Autodesk Fusion 360 part; units mm, degrees
note: some values were not read from the file. Chosen so that the rebuilt part matches the saved one: which bodies a step acts on; a direction; that a step has no effect; which face or edge a step refers to; which pieces of a blend or face edit are solid. Set by a fixed rule: which sketch regions a step uses.
(part 3 of 3)
chamfer "Fase5" distance 4 distance2 4.7 5 edges at (117, 33.2, 162.2) (55.5, 33.2, 162.2) (-2, 33.2, 162.2) (122, 87.4, 162.2) (-7, 87.4, 162.2) measured on face at (116.9689, 33.2, 167.6178) measured on face at (55.5311, 33.2, 167.6512) measured on face at (-1.9689, 33.2, 167.6178) measured on face at (122, 89.0667, 124.4667) measured on face at (-7, 85.7333, 101.1333) on bodies 16
chamfer "Fase6" distance 3 distance2 2.4 5 edges at (-2, 30.8, 202.2) (55.5, 30.8, 202.2) (117, 30.8, 202.2) (122, 87.4, 202.2) (-7, 87.4, 202.2) measured on face at (-3.6667, 30.8, 197.2) measured on face at (55.5311, 30.8, 195.1488) measured on face at (118.6667, 30.8, 197.2) measured on face at (122, 85.7333, 250.1333) measured on face at (-7, 85.7333, 284.4) on bodies 12
sketch "Skizze25" plane through (0, 0, -160.2) normal (0, 0, -1) x (-1, 0, 0)
  line L0 (9.4, 0) -> (9.4, 90)
  line L1 (-97.8, 90) -> (-185, 90)
  line L2 (-185, 90) -> (-185, 0)
  line L3 (-175, 47) -> (-1.2, 47)
  line L4 (-1.2, 47) -> (-1.2, 40)
  line L5 (-1.2, 40) -> (-175, 40)
  line L6 (-175, 40) -> (-175, 47)
  line L7 (-175, 50) -> (-1.2, 50)
  line L8 (-1.2, 50) -> (-1.2, 57)
  line L9 (-1.2, 57) -> (-175, 57)
  line L10 (-175, 57) -> (-175, 50)
  line L11 (-175, 60) -> (-1.2, 60)
  line L12 (-1.2, 60) -> (-1.2, 67)
  line L13 (-1.2, 67) -> (-175, 67)
  line L14 (-175, 67) -> (-175, 60)
  line L15 (-175, 70) -> (-1.2, 70)
  line L16 (-1.2, 70) -> (-1.2, 77)
  line L17 (-1.2, 77) -> (-175, 77)
  line L18 (-175, 77) -> (-175, 70)
  line L19 (-175, 80) -> (-1.2, 80)
  line L20 (-1.2, 80) -> (-1.2, 87)
  line L21 (-1.2, 87) -> (-175, 87)
  line L22 (-175, 87) -> (-175, 80)
  line L23 (-86.6, 87) -> (-89.6, 87)
  line L24 (-89.6, 87) -> (-89.6, 10)
  line L25 (-86.6, 10) -> (-86.6, 87)
  line L26 (8.8, 91.8) -> (8.8, 0)
  line L27 (-67.35, 22) -> (-50.9, 22)
  line L28 (-50.9, 22) -> (-50.9, 10)
  line L29 (-50.9, 10) -> (-67.35, 10)
  line L30 (-67.35, 10) -> (-67.35, 22)
  line L31 (-48.9, 10) -> (-48.9, 20)
  line L32 (-48.9, 20) -> (-31.68, 20)
  line L33 (-31.68, 20) -> (-31.68, 10)
  line L34 (-84.55, 10) -> (-84.55, 25)
  line L35 (-84.55, 25) -> (-69.35, 25)
  line L36 (-69.35, 25) -> (-69.35, 10)
  line L37 (-185, 0) -> (9.4, 0)
  line L38 (-175, 30) -> (-175, 37)
  line L39 (-1.2, 30) -> (-175, 30)
  line L40 (-84.55, 15) -> (-69.35, 15)
  line L41 (-175, 37) -> (-1.2, 37)
  line L42 (-1.2, 37) -> (-1.2, 30)
  line L43 (-89.6, 30) -> (-86.6, 30)
  line L44 (-175, 20) -> (-175, 27)
  line L45 (-1.2, 20) -> (-175, 20)
  line L46 (-84.55, 5) -> (-69.35, 5)
  line L47 (-175, 27) -> (-1.2, 27)
  line L48 (-1.2, 27) -> (-1.2, 20)
  line L49 (-89.6, 20) -> (-86.6, 20)
  line L50 (-175, 10) -> (-175, 17)
  line L51 (-1.2, 10) -> (-175, 10)
  line L52 (-84.55, -5) -> (-69.35, -5)
  line L53 (-175, 17) -> (-1.2, 17)
  line L54 (-1.2, 17) -> (-1.2, 10)
  line L55 (-89.6, 10) -> (-86.6, 10)
  line L56 (-56.3, 0) -> (-58.3, 0)
  line L57 (-58.3, 0) -> (-58.3, 47.5)
  line L58 (-58.3, 47.5) -> (-56.3, 47.5)
  line L59 (-56.3, 47.5) -> (-56.3, 0)
  line L60 (-58.3, 0) -> (-61.3, 0)
  line L61 (-61.3, 0) -> (-61.3, 47.5)
  line L62 (-61.3, 47.5) -> (-58.3, 47.5)
  line L63 (-58.3, 47.5) -> (-58.3, 0)
  line L64 (-56.3, 0) -> (-53.3, 0)
  line L65 (-53.3, 0) -> (-53.3, 49.9654)
  line L66 (-53.3, 49.9654) -> (-56.3, 49.9654)
  line L67 (-56.3, 49.9654) -> (-56.3, 0)
  line L68 (8.8, 0) -> (-122.3, 0)
  line L69 (-42.3, 57) -> (-42.3, 40)
  line L70 (-77.8, 90) -> (-77.8, 99)
  line L71 (-77.8, 99) -> (-84.8, 105)
  line L72 (-84.8, 105) -> (-90.8, 105)
  line L73 (-90.8, 105) -> (-97.8, 99)
  line L74 (-97.8, 99) -> (-97.8, 90)
  line L75 (9.4, 90) -> (-10.6, 90)
  line L76 (-10.6, 90) -> (-10.6, 99)
  line L77 (-10.6, 99) -> (-17.6, 105)
  line L78 (-17.6, 105) -> (-23.6, 105)
  line L79 (-23.6, 105) -> (-30.6, 99)
  line L80 (-30.6, 99) -> (-30.6, 90)
  line L81 (-30.6, 90) -> (-77.8, 90)
  line L82 (-31.68, 10) -> (-48.9, 10)
  line L83 (-69.35, 10) -> (-84.55, 10)
  circle A0 centre (-87.8, 99) radius 2.05
  circle A1 centre (-20.6, 99) radius 2.05
  point P0 (-57.3, 47.5)
  dimension "d531" = 7
  dimension "d533" = 7
  dimension "d534" = 7
  dimension "d535" = 7
  dimension "d536" = 3
  dimension "d537" = 3
  dimension "d538" = 3
  dimension "d539" = 7
  dimension "d540" = 3
  dimension "d541" = 10
  dimension "d561" = 3
  dimension "d719" = 10
  dimension "d720" = 7
  dimension "d721" = 7
  dimension "d722" = 7
  dimension "d723" = 3
  dimension "d724" = 3
  dimension "d725" = 3
  dimension "d726" = 2
  dimension "d727" = 3
  dimension "d728" = 3
  dimension "d753" = 15
  constraint horizontal L3
  constraint vertical L4
  constraint horizontal L5
  constraint vertical L6
  constraint horizontal L7
  constraint vertical L8
  constraint horizontal L9
  constraint vertical L10
  constraint horizontal L11
  constraint vertical L12
  constraint horizontal L13
  constraint vertical L14
  constraint horizontal L15
  constraint vertical L16
  constraint horizontal L17
  constraint vertical L18
  constraint horizontal L19
  constraint vertical L20
  constraint horizontal L21
  constraint vertical L22
  constraint vertical L3.start L7.start
  constraint vertical L9.end L11.start
  constraint vertical L13.end L15.start
  constraint vertical L3.end L7.end
  constraint vertical L8.end L11.end
  constraint vertical L12.end L15.end
  constraint vertical L16.end L19.end
  constraint horizontal L23
  constraint vertical L24
  constraint vertical L25
  constraint coincident L21 L23.end
  constraint vertical L17.end L19.start
  constraint horizontal L41
  constraint vertical L42
  constraint horizontal L39
  constraint vertical L38
  constraint horizontal L43
  constraint midpoint L39 L43
  constraint horizontal L47
  constraint vertical L48
  constraint horizontal L45
  constraint vertical L44
  constraint horizontal L49
  constraint midpoint L45 L49
  constraint horizontal L53
  constraint vertical L54
  constraint horizontal L51
  constraint vertical L50
  constraint horizontal L55
  constraint midpoint L51 L55
  constraint horizontal L56
  constraint vertical L57
  constraint horizontal L58
  constraint vertical L59
  constraint coincident L37 L56.start
  constraint midpoint L58 P0
  constraint horizontal L60
  constraint vertical L61
  constraint horizontal L62
  constraint vertical L63
  constraint horizontal L64
  constraint vertical L65
  constraint horizontal L66
  constraint vertical L67
  constraint vertical L5.end L38.end
  constraint vertical L38.start L44.end
  constraint vertical L44.start L50.end
  constraint coincident L34.start L51
  constraint coincident L9 L69.start
  constraint coincident L5 L69.end
  constraint perpendicular L5 L69
  measures "d531" distance of L3 L5
  measures "d533" distance of L7.start L9.end
  measures "d534" distance of L11.start L13.end
  measures "d535" distance of L15.start L17.end
  measures "d536" distance of L3 L7
  measures "d537" distance of L9 L11
  measures "d538" distance of L13 L15
  measures "d539" distance of L19.start L21.end
  measures "d540" distance of L17 L19
  measures "d541" distance of L2 L22
  measures "d561" distance of L24 L25
  measures "d719" distance of L20 L26
  measures "d720" distance of L39 L41
  measures "d721" distance of L45 L47
  measures "d722" distance of L51 L53
  measures "d723" distance of L5 L41
  measures "d724" distance of L39 L47
  measures "d725" distance of L45 L53
  measures "d726" distance of L57 L59
  measures "d727" distance of L56.end L60.end
  measures "d728" distance of L56.start L64.end
  measures "d753" distance of P0 L69
sketch "Skizze26" plane through (-9.4, 0, 0) normal (-1, 0, 0) x (0, 0, 1)
  line L0 (-69.4, 90) -> (-120.2, 90)
  line L1 (-120.2, 90) -> (-120.2, 98)
  line L2 (-126.2, 105) -> (-134.2, 105)
  line L3 (-150.2, 47) -> (-39.4, 47)
  line L4 (-39.4, 47) -> (-39.4, 40)
  line L5 (-39.4, 40) -> (-150.2, 40)
  line L6 (-150.2, 40) -> (-150.2, 47)
  line L7 (-150.2, 50) -> (-39.4, 50)
  line L8 (-39.4, 50) -> (-39.4, 57)
  line L9 (-39.4, 57) -> (-150.2, 57)
  line L10 (-150.2, 57) -> (-150.2, 50)
  line L11 (-150.2, 60) -> (-39.4, 60)
  line L12 (-39.4, 60) -> (-39.4, 67)
  line L13 (-39.4, 67) -> (-150.2, 67)
  line L14 (-150.2, 67) -> (-150.2, 60)
  line L15 (-150.2, 70) -> (-39.4, 70)
  line L16 (-39.4, 70) -> (-39.4, 77)
  line L17 (-39.4, 77) -> (-150.2, 77)
  line L18 (-150.2, 77) -> (-150.2, 70)
  line L19 (-150.2, 87) -> (-39.4, 87)
  line L20 (-39.4, 87) -> (-39.4, 80)
  line L21 (-39.4, 80) -> (-150.2, 80)
  line L22 (-150.2, 80) -> (-150.2, 87)
  line L23 (-150.2, 37) -> (-39.4, 37)
  line L24 (-39.4, 37) -> (-39.4, 30)
  line L25 (-39.4, 30) -> (-150.2, 30)
  line L26 (-150.2, 30) -> (-150.2, 37)
  line L27 (-150.2, 27) -> (-39.4, 27)
  line L28 (-39.4, 27) -> (-39.4, 20)
  line L29 (-39.4, 20) -> (-150.2, 20)
  line L30 (-150.2, 20) -> (-150.2, 27)
  line L31 (-96.3, 87) -> (-93.3, 87)
  line L32 (-93.3, 87) -> (-93.3, 10)
  line L33 (-93.3, 10) -> (-96.3, 10)
  line L34 (-96.3, 10) -> (-96.3, 87)
  line L35 (-29.4, 185.4469) -> (-29.4, 23.7878)
  line L36 (-150.2, 17) -> (-39.4, 17)
  line L37 (-39.4, 10) -> (-150.2, 10)
  line L38 (-39.4, 17) -> (-39.4, 10)
  line L39 (-150.2, 10) -> (-150.2, 17)
  line L40 (-131.2, 38.5) -> (-129.2, 38.5)
  line L41 (-129.2, 38.5) -> (-129.2, 0)
  line L42 (-129.2, 0) -> (-131.2, 0)
  line L43 (-131.2, 0) -> (-131.2, 38.5)
  line L44 (-60.4, 0) -> (-58.4, 0)
  line L45 (-58.4, 0) -> (-58.4, 38.5)
  line L46 (-58.4, 38.5) -> (-60.4, 38.5)
  line L47 (-60.4, 38.5) -> (-60.4, 0)
  line L48 (-60.4, 38.5) -> (-63.4, 38.5)
  line L49 (-63.4, 38.5) -> (-63.4, 10)
  line L50 (-63.4, 10) -> (-60.4, 10)
  line L51 (-60.4, 10) -> (-60.4, 38.5)
  line L52 (-58.4, 38.5) -> (-55.4, 38.5)
  line L53 (-55.4, 38.5) -> (-55.4, 10)
  line L54 (-58.4, 0) -> (-58.4, 38.5)
  line L55 (-160.2, 0) -> (-160.2, 90)
  line L56 (-29.4, 0) -> (-160.2, 0)
  line L57 (-129.2, 38.5) -> (-126.2, 38.5)
  line L58 (-126.2, 38.5) -> (-126.2, 10)
  line L59 (-126.2, 10) -> (-129.2, 10)
  line L60 (-129.2, 10) -> (-129.2, 38.5)
  line L61 (-131.2, 38.5) -> (-134.2, 38.5)
  line L62 (-134.2, 38.5) -> (-134.2, 10)
  line L63 (-134.2, 10) -> (-131.2, 10)
  line L64 (-131.2, 10) -> (-131.2, 38.5)
  line L65 (-74.4, 47) -> (-113.2155, 47)
  line L66 (-113.2155, 47) -> (-113.2155, 30)
  line L67 (-113.2155, 30) -> (-74.4, 30)
  line L68 (-74.4, 30) -> (-74.4, 47)
  circle A0 centre (-59.4, 38.5) radius 10
  line L69 (-134.2, 105) -> (-140.2, 98)
  line L70 (-49.4, 98) -> (-55.4, 105)
  line L71 (-63.4, 105) -> (-69.4, 98)
  line L72 (-120.2, 98) -> (-126.2, 105)
  line L73 (-29.4, 90) -> (-49.4, 90)
  line L74 (-29.4, 0) -> (-29.4, 90)
  line L75 (-69.4, 98) -> (-69.4, 90)
  circle A1 centre (-130.2, 99) radius 2.05
  point P0 (-130.2, 38.5)
  point P1 (-59.4, 38.5)
  dimension "d542" = 7
  dimension "d545" = 7
  dimension "d546" = 7
  dimension "d547" = 7
  dimension "d548" = 3
  dimension "d549" = 3
  dimension "d550" = 3
  dimension "d551" = 7
  dimension "d552" = 3
  dimension "d553" = 7
  dimension "d556" = 3
  dimension "d557" = 3
  dimension "d559" = 7
  dimension "d560" = 3
  dimension "d730" = 10
  dimension "d731" = 7
  dimension "d732" = 3
  dimension "d738" = 2
  dimension "d739" = 2
  dimension "d741" = 3
  dimension "d743" = 3
  dimension "d744" = 10
  dimension "d745" = 10
  dimension "d749" = 3
  dimension "d750" = 3
  dimension "d751" = 15
  dimension "d752" = 16.9845
  constraint horizontal L3
  constraint vertical L4
  constraint horizontal L5
  constraint vertical L6
  constraint horizontal L7
  constraint vertical L8
  constraint horizontal L9
  constraint vertical L10
  constraint horizontal L11
  constraint vertical L12
  constraint horizontal L13
  constraint vertical L14
  constraint horizontal L15
  constraint vertical L16
  constraint horizontal L17
  constraint vertical L18
  constraint horizontal L19
  constraint vertical L20
  constraint horizontal L21
  constraint vertical L22
  constraint vertical L3.start L7.start
  constraint vertical L9.end L11.start
  constraint vertical L13.end L15.start
  constraint vertical L17.end L21.end
  constraint vertical L3.end L7.end
  constraint vertical L8.end L11.end
  constraint vertical L12.end L15.end
  constraint vertical L16.end L20.end
  constraint horizontal L23
  constraint vertical L24
  constraint horizontal L25
  constraint vertical L26
  constraint horizontal L27
  constraint vertical L28
  constraint horizontal L29
  constraint vertical L30
  constraint vertical L5.end L23.start
  constraint vertical L25.end L27.start
  constraint vertical L24.end L27.end
  constraint vertical L4.end L23.end
  constraint horizontal L31
  constraint vertical L32
  constraint horizontal L33
  constraint vertical L34
  constraint coincident L19 L31.start
  constraint midpoint L19 L31
  constraint horizontal L36
  constraint vertical L38
  constraint horizontal L37
  constraint vertical L39
  constraint coincident L32.end L37
  constraint vertical L29.end L36.start
  constraint vertical L28.end L36.end
  constraint horizontal L40
  constraint vertical L41
  constraint horizontal L42
  constraint vertical L43
  constraint midpoint L40 P0
  constraint horizontal L44
  constraint vertical L45
  constraint horizontal L46
  constraint vertical L47
  constraint midpoint L46 P1
  constraint horizontal L48
  constraint vertical L49
  constraint horizontal L50
  constraint vertical L51
  constraint horizontal L52
  constraint vertical L53
  constraint vertical L54
  constraint coincident L37 L53.end
  constraint coincident L37 L49.end
  constraint horizontal L57
  constraint vertical L58
  constraint horizontal L59
  constraint vertical L60
  constraint horizontal L61
  constraint vertical L62
  constraint horizontal L63
  constraint vertical L64
  constraint coincident L37 L62.end
  constraint coincident L37 L58.end
  constraint horizontal L65
  constraint vertical L66
  constraint horizontal L67
  constraint vertical L68
  constraint coincident L25 L66.end
  constraint coincident L3 L65.start
  constraint coincident L44.end L56
  constraint coincident L44.start L56
  constraint coincident L41.end L56
  measures "d542" distance of L3.start L5.end
  measures "d545" distance of L7.start L9.end
  measures "d546" distance of L11.start L13.end
  measures "d547" distance of L15.start L17.end
  measures "d548" distance of L3 L7
  measures "d549" distance of L9 L11
  measures "d550" distance of L13 L15.end
  measures "d551" distance of L19.start L21.end
  measures "d552" distance of L17 L21
  measures "d553" distance of L23.start L25.end
  measures "d556" distance of L5 L23
  measures "d557" distance of L25 L27
  measures "d559" distance of L27 L29
  measures "d560" distance of L32 L34
  measures "d730" distance of L20 L35
  measures "d731" distance of L36 L37
  measures "d732" distance of L29 L36
  measures "d738" distance of L41 L43
  measures "d739" distance of L45 L47
  measures "d741" distance of L46.end L48.end
  measures "d743" distance of L45.end L52.end
  measures "d744" distance of L22 L55
  measures "d745" distance of L37 L56
  measures "d749" distance of L40.end L57.end
  measures "d750" distance of L40.start L61.end
  measures "d751" distance of L68 P1
  measures "d752" distance of P0 L66
sketch "Skizze27" plane through (0, -2.4, 0) normal (0, -1, 0) x (-1, 0, 0)
  line L0 (-29.653, 141.5068) -> (-29.653, 45.5068)
  line L1 (-29.653, 45.5068) -> (-36.653, 45.5068)
  line L2 (-36.653, 141.5068) -> (-29.653, 141.5068)
  line L3 (-66.653, 45.5068) -> (-66.653, 141.5068)
  line L4 (-59.653, 45.5068) -> (-66.653, 45.5068)
  line L5 (-69.653, 45.5068) -> (-76.653, 45.5068)
  line L6 (-39.653, 45.5068) -> (-46.653, 45.5068)
  line L7 (-49.653, 45.5068) -> (-56.653, 45.5068)
  line L8 (-39.653, 141.5068) -> (-39.653, 45.5068)
  line L9 (-59.653, 141.5068) -> (-59.653, 45.5068)
  line L10 (-46.653, 45.5068) -> (-46.653, 141.5068)
  line L11 (-56.653, 45.5068) -> (-56.653, 141.5068)
  line L12 (-69.653, 141.5068) -> (-69.653, 45.5068)
  line L13 (-49.653, 141.5068) -> (-49.653, 45.5068)
  line L14 (-76.653, 45.5068) -> (-76.653, 141.5068)
  line L15 (-46.653, 141.5068) -> (-39.653, 141.5068)
  line L16 (-66.653, 141.5068) -> (-59.653, 141.5068)
  line L17 (-76.653, 141.5068) -> (-69.653, 141.5068)
  line L18 (-56.653, 141.5068) -> (-49.653, 141.5068)
  line L19 (-106.653, 45.5068) -> (-106.653, 141.5068)
  line L20 (-99.653, 45.5068) -> (-106.653, 45.5068)
  line L21 (-109.653, 45.5068) -> (-116.653, 45.5068)
  line L22 (-79.653, 45.5068) -> (-86.653, 45.5068)
  line L23 (-89.653, 45.5068) -> (-96.653, 45.5068)
  line L24 (-79.653, 141.5068) -> (-79.653, 45.5068)
  line L25 (-99.653, 141.5068) -> (-99.653, 45.5068)
  line L26 (-86.653, 45.5068) -> (-86.653, 141.5068)
  line L27 (-96.653, 45.5068) -> (-96.653, 141.5068)
  line L28 (-109.653, 141.5068) -> (-109.653, 45.5068)
  line L29 (-89.653, 141.5068) -> (-89.653, 45.5068)
  line L30 (-116.653, 45.5068) -> (-116.653, 141.5068)
  line L31 (-86.653, 141.5068) -> (-79.653, 141.5068)
  line L32 (-106.653, 141.5068) -> (-99.653, 141.5068)
  line L33 (-116.653, 141.5068) -> (-109.653, 141.5068)
  line L34 (-96.653, 141.5068) -> (-89.653, 141.5068)
  line L35 (-146.653, 45.5068) -> (-146.653, 141.5068)
  line L36 (-139.653, 45.5068) -> (-146.653, 45.5068)
  line L37 (-161.653, 45.5068) -> (-168.653, 45.5068)
  line L38 (-119.653, 45.5068) -> (-126.653, 45.5068)
  line L39 (-129.653, 45.5068) -> (-136.653, 45.5068)
  line L40 (-119.653, 141.5068) -> (-119.653, 45.5068)
  line L41 (-139.653, 141.5068) -> (-139.653, 45.5068)
  line L42 (-126.653, 45.5068) -> (-126.653, 141.5068)
  line L43 (-136.653, 45.5068) -> (-136.653, 141.5068)
  line L44 (-161.653, 141.5068) -> (-161.653, 45.5068)
  line L45 (-129.653, 141.5068) -> (-129.653, 45.5068)
  line L46 (-168.653, 45.5068) -> (-168.653, 141.5068)
  line L47 (-126.653, 141.5068) -> (-119.653, 141.5068)
  line L48 (-146.653, 141.5068) -> (-139.653, 141.5068)
  line L49 (-168.653, 141.5068) -> (-161.653, 141.5068)
  line L50 (-136.653, 141.5068) -> (-129.653, 141.5068)
  line L51 (-36.653, 45.5068) -> (-36.653, 141.5068)
  line L52 (-178.653, 45.5068) -> (-178.653, 141.5068)
  line L53 (-171.653, 45.5068) -> (-178.653, 45.5068)
  line L54 (-171.653, 141.5068) -> (-171.653, 45.5068)
  line L55 (-178.653, 141.5068) -> (-171.653, 141.5068)
  line L56 (-29.653, 95.0068) -> (-29.653, 92.0068)
  line L57 (-29.653, 92.0068) -> (-178.653, 92.0068)
  line L58 (-178.653, 92.0068) -> (-178.653, 95.0068)
  line L59 (-178.653, 95.0068) -> (-29.653, 95.0068)
  circle A0 centre (-179.1, 154.3) radius 1.5
  circle A1 centre (3.5, 35.3) radius 1.5
  circle A2 centre (-155.5, 66.3) radius 1.5
  circle A3 centre (-17.5, 66.3) radius 1.5
  circle A4 centre (-179.1, 35.3) radius 1.5
  line L60 (2, 96.8) -> (-8, 96.8)
  line L61 (-8, 96.8) -> (-8, 116.8)
  line L62 (-8, 116.8) -> (2, 116.8)
  line L63 (2, 116.8) -> (2, 96.8)
  circle A5 centre (-17.5, 152.3) radius 1.5
  circle A6 centre (-155.5, 152.3) radius 1.5
  circle A7 centre (3.5, 154.3) radius 1.5
  line L64 (-185, 29.4) -> (9.4, 29.4)
  line L65 (9.4, 29.4) -> (9.4, 160.2)
  line L66 (9.4, 160.2) -> (-185, 160.2)
  line L67 (-185, 160.2) -> (-185, 29.4)
  line L68 (-97.8, 157.8) -> (-182.6, 157.8)
  line L69 (-30.6, 157.8) -> (-77.8, 157.8)
  line L70 (7, 157.8) -> (-10.6, 157.8)
  point P0 (-36.653, 141.5068)
  point P1 (-36.653, 45.5068)
  point P2 (-36.653, 141.5068)
  point P3 (-79.653, 143.3514)
  point P4 (-76.653, 45.5068)
  point P5 (-76.653, 144.8311)
  dimension "d573" = 7
  dimension "d583" = 7
  dimension "d584" = 7
  dimension "d585" = 7
  dimension "d587" = 3
  dimension "d588" = 3
  dimension "d589" = 3
  dimension "d591" = 7
  dimension "d592" = 7
  dimension "d593" = 7
  dimension "d594" = 3
  dimension "d595" = 3
  dimension "d596" = 3
  dimension "d597" = 7
  dimension "d598" = 7
  dimension "d599" = 7
  dimension "d600" = 7
  dimension "d601" = 3
  dimension "d602" = 3
  dimension "d603" = 15
  dimension "d604" = 3
  dimension "d607" = 3
  dimension "d608" = 7
  dimension "d609" = 7
  dimension "d611" = 3
  dimension "d612" = 7
  dimension "d613" = 3
  dimension "d614" = 3
  constraint coincident P2 P0
  constraint coincident P1 L1.end
  constraint perpendicular L1 L51
  constraint midpoint L52 L58
  constraint coincident L0 L56.end
  measures "d573" distance of L0.start P2
  measures "d583" distance of L10.end L8.start
  measures "d584" distance of L13.start L11.end
  measures "d585" distance of L9.start L3.end
  measures "d587" distance of L10 L13
  measures "d588" distance of L9 L11
  measures "d589" distance of L3 L12
  measures "d591" distance of L29.start L27.end
  measures "d592" distance of L25.start L19.end
  measures "d593" distance of L28.start L30.end
  measures "d594" distance of L26 L29
  measures "d595" distance of L25 L27
  measures "d596" distance of L19 L28
  measures "d597" distance of L42.end L40.start
  measures "d598" distance of L45.start L43.end
  measures "d599" distance of L41.start L35.end
  measures "d600" distance of L44.start L46.end
  measures "d601" distance of L42 L45
  measures "d602" distance of L41 L43
  measures "d603" distance of L35 L44
  measures "d604" distance of L14 L24
  measures "d607" distance of L8 L51
  measures "d608" distance of L12 L14
  measures "d609" distance of L24 L26
  measures "d611" distance of L30 L40
  measures "d612" distance of L54.start L52.end
  measures "d613" distance of L46 L54
  measures "d614" distance of L57.end L58.end
extrude "Extrusion49" cut sketch "Skizze25" against normal up to surface (2.4 mm away) contours L39 L41 L42 L65 | L39 L41 L59 L65 L67 | L39 L41 L57 L59 L63 L67 | L39 L41 L57 L61 L63 | L3 L5 L65 L69 | L3 L5 L59 L65 L67 | L24 L50 L51 L53 | L25 L39 L41 L61 | L3 L5 L57 L59 L63 L67 | L3 L4 L5 L69 | L24 L44 L45 L47 | L3 L5 L57 L61 L63 | L24 L38 L39 L41 | L3 L5 L25 L61 | L7 L8 L9 L69 | L7 L9 L25 L69 | L3 L5 L6 L24 | L7 L9 L10 L24 | L11 L12 L13 L25 | L11 L13 L14 L24 | L15 L16 L17 L25 | L15 L17 L18 L24 | L19 L20 L21 L25 | L19 L21 L22 L24 bodies 5
extrude "Extrusion50" cut sketch "Skizze26" against normal up to surface (2.4 mm away) contours L3 L5 L6 L66 | L3 L5 L34 L65 L66 | L3 L5 L32 L65 L68 | L7 L9 L10 L34 | L23 L25 L58 L66 | L23 L25 L34 L66 L67 | L3 L5 L68 A0 | L7 L8 L9 L32 | L23 L25 L41 L58 L60 | L3 L5 A0 | L23 L25 L32 L67 L68 | L11 L13 L14 L34 | L23 L25 L41 L43 L60 L64 | L3 L4 L5 A0 | L23 L25 L68 A0 | L11 L12 L13 L32 | L27 L29 L34 L58 | L23 L25 L43 L62 L64 | L27 L29 L41 L58 L60 | L23 L25 L49 A0 | L27 L29 L32 L49 | L15 L17 L18 L34 | L23 L25 L26 L62 | L27 L29 L41 L43 L60 L64 | L23 L25 L47 L49 L51 | L15 L16 L17 L32 | L27 L29 L47 L49 L51 | L34 L36 L37 L58 | L27 L29 L43 L62 L64 | L36 L37 L41 L58 L59 L60 | L23 L25 L53 A0 | L23 L24 L25 A0 | L23 L25 L45 L47 L51 L54 | L27 L29 L45 L47 L51 L54 | L32 L36 L37 L49 | L19 L21 L22 L34 | L27 L29 L30 L62 | L36 L37 L41 L43 L60 L64 | L23 L25 L45 L53 L54 | L19 L20 L21 L32 | L27 L29 L45 L53 L54 | L36 L37 L47 L49 L50 L51 | L36 L37 L43 L62 L63 L64 | L27 L28 L29 L53 | L36 L37 L45 L47 L51 L54 | L36 L37 L39 L62 | L36 L37 L45 L53 L54 | L36 L37 L38 L53 bodies 5
extrude "Extrusion63" cut sketch "Skizze25" along normal up to surface (2.4 mm away) from surface at -130.8 contours L29 L37 L51 L56 L57 L59 L63 L67 L68 | L28 L29 L51 L53 L65 | L29 L51 L53 L57 L59 L63 L67 | L28 L31 L51 L53 | L45 L53 L57 L59 L63 L67 | L31 L33 L51 L53 L82 | L27 L28 L45 L65 | L29 L30 L51 L53 L61 | L27 L45 L57 L59 L63 L67 | L27 L28 L32 L45 L47 L48 L65 | L33 L51 L53 L54 | L30 L36 L51 L53 | L27 L47 L57 L59 L63 L67 | L34 L36 L40 L51 L83 | L27 L30 L45 L61 | L39 L47 L57 L59 L63 L67 | L39 L41 L42 L65 | L25 L27 L30 L34 L35 L36 L45 L47 L61 | L34 L36 L40 L53 | L25 L34 L51 L53 | L39 L41 L57 L59 L63 L67 | L34 L35 L36 L45 | L5 L41 L57 L59 L63 L67 | L24 L50 L51 L53 | L25 L39 L41 L61 | L3 L5 L57 L59 L63 L67 | L3 L4 L5 L69 | L24 L44 L45 L47 | L24 L38 L39 L41 | L7 L8 L9 L69 | L3 L5 L6 L24 | L7 L9 L10 L24 | L11 L12 L13 L25 | L11 L13 L14 L24 | L15 L16 L17 L25 | L15 L17 L18 L24 bodies 5
extrude "Extrusion64" cut sketch "Skizze26" against normal up to surface (2.4 mm away) from surface at -192 contours L3 L5 L34 L65 L66 | L3 L5 L32 L65 L68 | L7 L9 L10 L34 | L23 L25 L34 L66 L67 | L7 L8 L9 L32 | L23 L25 L32 L67 L68 | L11 L13 L14 L34 | L23 L25 L41 L43 L60 L64 | L11 L12 L13 L32 | L27 L29 L34 L58 | L25 L27 L41 L43 L60 L64 | L27 L29 L32 L49 | L15 L17 L18 L34 | L27 L29 L41 L43 L60 L64 | L15 L16 L17 L32 | L34 L36 L37 L58 | L29 L36 L41 L43 L60 L64 | L23 L25 L45 L47 L51 L54 | L27 L45 L47 L51 L54 A0 | L27 L29 L45 L47 L51 L54 | L32 L36 L37 L49 | L19 L21 L22 L34 | L27 L29 L30 L62 | L36 L37 L41 L43 L60 L64 | L25 L45 L47 L51 L54 A0 | L19 L20 L21 L32 | L29 L36 L45 L47 L51 L54 | L37 L41 L42 L43 L56 | L27 L28 L29 L53 | L36 L37 L45 L47 L51 L54 | L36 L37 L39 L62 | L37 L44 L45 L47 L54 L56 | L36 L37 L38 L53 bodies 5
extrude "Extrusion52" cut sketch "Skizze27" against normal up to surface (2.4 mm away) contours L0 L2 L51 L59 | L0 L1 L51 L57 | L8 L10 L15 L59 | L6 L8 L10 L57 | L11 L13 L18 L59 | L7 L11 L13 L57 | L3 L9 L16 L59 | L3 L4 L9 L57 | L12 L14 L17 L59 | L5 L12 L14 L57 | L24 L26 L31 L59 | L22 L24 L26 L57 | L27 L29 L34 L59 | L23 L27 L29 L57 | L19 L25 L32 L59 | L19 L20 L25 L57 | L28 L30 L33 L59 | L21 L28 L30 L57 | L40 L42 L47 L59 | L38 L40 L42 L57 | L43 L45 L50 L59 | L39 L43 L45 L57 | L35 L41 L48 L59 | L35 L36 L41 L57 | L44 L46 L49 L59 | L52 L54 L55 L59 | L52 L53 L54 L57 bodies 2 3 4 7 5 8 10 11 12 16 28
hidden bodies 5 4 7 10 11
equation "d1 = PSULänge"
equation "d2 = PSUBreite"
equation "PSULänge = 240 mm"
equation "PSUBreite = 115 mm"
equation "PSUHöhe = 50 mm"
equation "PSULüftungsabstand = 7 mm"
equation "d7 = PSULüftungsabstand"
equation "d8 = PSULüftungsabstand"
equation "d9 = PSULüftungsabstand"
equation "Wandstärke = 2.4 mm"
equation "d12 = Wandstärke"
equation "d13 = WandstärkeDick"
equation "d14 = Wandstärke"
equation "d15 = Wandstärke"
equation "d16 = Wandstärke"
equation "d18 = PSUHöhe + PSULüftungsabstand * 2"
equation "WandstärkeDick = 4 mm"
equation "SteckerAbstand = 50 mm"
equation "d24 = SteckerAbstand"
equation "d41 = PSUHöhe"
equation "PSULängeReal = 215 mm"
equation "d61 = PSULängeReal"
equation "d69 = PSUSchraubenDM"
equation "d70 = PSUSchraubenDM"
equation "PSUSchraubenDM = 3.7 mm"
equation "d82 = -( PSULüftungsabstand - 1 mm )"
equation "d85 = PSULüftungsabstand - 1 mm"
equation "d89 = 30 mm + 10 mm"
equation "d90 = Wandstärke"
equation "AufhängungLochDM = 4.1 mm"
equation "d128 = AufhängungLochDM"
equation "d131 = AufhängungLochDM"
equation "d134 = AufhängungLochDM"
equation "d139 = AufhängungLochDM"
equation "d146 = AufhängungLochDM"
equation "d158 = Wandstärke"
equation "d159 = Wandstärke"
equation "d160 = Wandstärke"
equation "d161 = Wandstärke"
equation "d171 = SKRBoardLochDM"
equation "SKRBoardLochDM = 3 mm"
equation "d173 = SKRBoardLochDM"
equation "d174 = SKRBoardLochDM"
equation "d175 = SKRBoardLochDM"
equation "d180 = ( 91.65 mm - 75.45 mm )"
equation "d183 = 110.1 mm - 91.65 mm"
equation "d188 = -Wandstärke"
equation "d190 = Wandstärke"
equation "d191 = Wandstärke"
equation "d192 = Wandstärke"
equation "d193 = Wandstärke"
equation "d232 = 128.32 mm - 110.10 mm"
equation "d290 = AufhängungLochDM"
equation "d300 = AufhängungLochDM"
equation "d398 = ( 27.5 mm - 16.5 mm ) / 2"
equation "d406 = Wandstärke"
equation "d410 = 2 * Wandstärke"
equation "d413 = Wandstärke"
equation "d426 = PSUBreite / 2"
equation "d444 = Wandstärke"
equation "d445 = Wandstärke"
equation "d446 = Wandstärke"
equation "d448 = Wandstärke"
equation "d449 = -Wandstärke"
equation "d457 = Wandstärke"
equation "d466 = 2 * Wandstärke"
equation "d469 = Wandstärke"
equation "d472 = -Wandstärke"
equation "d475 = -2 * Wandstärke"
equation "d478 = -Wandstärke"
equation "d635 = SKRBoardLochDM"
equation "d638 = SKRBoardLochDM"
equation "d640 = SKRBoardLochDM"
equation "d642 = SKRBoardLochDM"
equation "d689 = AufhängungLochDM"
equation "d694 = AufhängungLochDM"
equation "d713 = Wandstärke"
equation "d714 = Wandstärke"
equation "d715 = Wandstärke"
equation "d716 = Wandstärke"
equation "d768 = Wandstärke"
named bodies: "PSU-Gehäuse", "PSU", "PSU-Gehäuse-Deckel", "SKR-Gehäuseboden", "SKR-Platzhalter", "120mm Fan", "PSU-Gehäuse 2", "PSU-Gehäuse-Deckel (1)", "PSU-Gehäuse (1)", "SKR Fan-Abdeckung", "SKR-Gehäusewände", "SKR-Gehäusedeckel"
